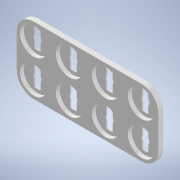
# Autodesk Inventor part: Деталь4
Saved by Autodesk Inventor 2020 (Build 240168000, 168)
## iProperties
Created: 2023-05-30
Part Number: Деталь4
Material: Типовые
Document SubType Name: Modeling
Designer: Qwellert
Density: 1 g/cm^3
Appearance: По умолчанию
Author: Qwellert
Autodesk Inventor part; units mm, degrees
ref_plane "YZ Plane" through (0, 0, 0) normal (1, 0, 0) x (0, 1, 0)
ref_plane "XZ Plane" through (0, 0, 0) normal (0, 1, 0) x (-1, 0, 0)
ref_plane "XY Plane" through (0, 0, 0) normal (0, 0, 1) x (1, 0, 0)
sketch "Эскиз1" plane through (0, 0, 0) normal (0, 0, 1) x (1, 0, 0)
  circle A0 centre (0, 0) radius 13.8038 projected
  arc A1 (3.05, 9.7271) -> (-3.05, 9.7271) centre (0, 0) ccw projected
  line L0 (3.05, 9.7271) -> (3.05, 2.51) projected
  arc A2 (3.05, -2.51) -> (3.05, 2.51) centre (0, 0) ccw projected
  line L1 (3.05, -2.51) -> (3.05, -9.7271) projected
  arc A3 (-3.05, -9.7271) -> (3.05, -9.7271) centre (0, 0) ccw projected
  line L2 (-3.05, -9.7271) -> (-3.05, -2.51) projected
  arc A4 (-3.05, 2.51) -> (-3.05, -2.51) centre (0, 0) ccw projected
  line L3 (-3.05, 2.51) -> (-3.05, 9.7271) projected
  arc A5 (-3.05, 2.51) -> (-3.05, -2.51) centre (0, 0) ccw
  line L4 (-3.05, -2.51) -> (-3.05, -9.7271)
  arc A6 (-3.05, -9.7271) -> (3.05, -9.7271) centre (0, 0) ccw
  line L5 (3.05, -9.7271) -> (3.05, -2.51)
  arc A7 (3.05, -2.51) -> (3.05, 2.51) centre (0, 0) ccw
  line L6 (3.05, 2.51) -> (3.05, 9.7271)
  arc A8 (3.05, 9.7271) -> (-3.05, 9.7271) centre (0, 0) ccw
  line L7 (-3.05, 9.7271) -> (-3.05, 2.51)
  circle A9 centre (0, 0) radius 13.8038
  arc A10 (-3.05, -31.3679) -> (-3.05, -36.3879) centre (0, -33.8779) ccw
  line L8 (-3.05, -36.3879) -> (-3.05, -43.605)
  arc A11 (-3.05, -43.605) -> (3.05, -43.605) centre (0, -33.8779) ccw
  line L9 (3.05, -43.605) -> (3.05, -36.3879)
  arc A12 (3.05, -36.3879) -> (3.05, -31.3679) centre (0, -33.8779) ccw
  line L10 (3.05, -31.3679) -> (3.05, -24.1507)
  arc A13 (3.05, -24.1507) -> (-3.05, -24.1507) centre (0, -33.8779) ccw
  line L11 (-3.05, -24.1507) -> (-3.05, -31.3679)
  circle A14 centre (0, -33.8779) radius 13.8038
  arc A15 (-39.3128, 2.51) -> (-39.3128, -2.51) centre (-36.2628, 0) ccw
  line L12 (-39.3128, -2.51) -> (-39.3128, -9.7271)
  arc A16 (-39.3128, -9.7271) -> (-33.2128, -9.7271) centre (-36.2628, 0) ccw
  line L13 (-33.2128, -9.7271) -> (-33.2128, -2.51)
  arc A17 (-33.2128, -2.51) -> (-33.2128, 2.51) centre (-36.2628, 0) ccw
  line L14 (-33.2128, 2.51) -> (-33.2128, 9.7271)
  arc A18 (-33.2128, 9.7271) -> (-39.3128, 9.7271) centre (-36.2628, 0) ccw
  line L15 (-39.3128, 9.7271) -> (-39.3128, 2.51)
  circle A19 centre (-36.2628, 0) radius 13.8038
  circle A20 centre (-36.2628, -33.8779) radius 13.8038
  line L16 (-33.2128, -43.605) -> (-33.2128, -36.3879)
  arc A21 (-39.3128, -43.605) -> (-33.2128, -43.605) centre (-36.2628, -33.8779) ccw
  line L17 (-39.3128, -36.3879) -> (-39.3128, -43.605)
  arc A22 (-39.3128, -31.3679) -> (-39.3128, -36.3879) centre (-36.2628, -33.8779) ccw
  arc A23 (-33.2128, -36.3879) -> (-33.2128, -31.3679) centre (-36.2628, -33.8779) ccw
  line L18 (-33.2128, -31.3679) -> (-33.2128, -24.1507)
  arc A24 (-33.2128, -24.1507) -> (-39.3128, -24.1507) centre (-36.2628, -33.8779) ccw
  line L19 (-39.3128, -24.1507) -> (-39.3128, -31.3679)
  arc A25 (-75.5758, 2.51) -> (-75.5758, -2.51) centre (-72.5258, 0) ccw
  line L20 (-75.5758, -2.51) -> (-75.5758, -9.7271)
  arc A26 (-75.5758, -9.7271) -> (-69.4758, -9.7271) centre (-72.5258, 0) ccw
  line L21 (-69.4758, -9.7271) -> (-69.4758, -2.51)
  arc A27 (-69.4758, -2.51) -> (-69.4758, 2.51) centre (-72.5258, 0) ccw
  line L22 (-69.4758, 2.51) -> (-69.4758, 9.7271)
  arc A28 (-69.4758, 9.7271) -> (-75.5758, 9.7271) centre (-72.5258, 0) ccw
  line L23 (-75.5758, 9.7271) -> (-75.5758, 2.51)
  circle A29 centre (-72.5258, 0) radius 13.8038
  circle A30 centre (-72.5258, -33.8779) radius 13.8038
  line L24 (-69.4758, -43.605) -> (-69.4758, -36.3879)
  arc A31 (-75.5758, -43.605) -> (-69.4758, -43.605) centre (-72.5258, -33.8779) ccw
  line L25 (-75.5758, -36.3879) -> (-75.5758, -43.605)
  arc A32 (-75.5758, -31.3679) -> (-75.5758, -36.3879) centre (-72.5258, -33.8779) ccw
  arc A33 (-69.4758, -36.3879) -> (-69.4758, -31.3679) centre (-72.5258, -33.8779) ccw
  line L26 (-69.4758, -31.3679) -> (-69.4758, -24.1507)
  arc A34 (-69.4758, -24.1507) -> (-75.5758, -24.1507) centre (-72.5258, -33.8779) ccw
  line L27 (-75.5758, -24.1507) -> (-75.5758, -31.3679)
  circle A35 centre (-108.7886, 0) radius 13.8038
  line L28 (-105.7386, -9.7271) -> (-105.7386, -2.51)
  arc A36 (-111.8386, -9.7271) -> (-105.7386, -9.7271) centre (-108.7886, 0) ccw
  line L29 (-111.8386, -2.51) -> (-111.8386, -9.7271)
  arc A37 (-111.8386, 2.51) -> (-111.8386, -2.51) centre (-108.7886, 0) ccw
  arc A38 (-105.7386, -2.51) -> (-105.7386, 2.51) centre (-108.7886, 0) ccw
  line L30 (-105.7386, 2.51) -> (-105.7386, 9.7271)
  arc A39 (-105.7386, 9.7271) -> (-111.8386, 9.7271) centre (-108.7886, 0) ccw
  line L31 (-111.8386, 9.7271) -> (-111.8386, 2.51)
  circle A40 centre (-108.7886, -33.8779) radius 13.8038
  line L32 (-105.7386, -31.3679) -> (-105.7386, -24.1507)
  arc A41 (-105.7386, -36.3879) -> (-105.7386, -31.3679) centre (-108.7886, -33.8779) ccw
  line L33 (-105.7386, -43.605) -> (-105.7386, -36.3879)
  arc A42 (-111.8386, -43.605) -> (-105.7386, -43.605) centre (-108.7886, -33.8779) ccw
  line L34 (-111.8386, -36.3879) -> (-111.8386, -43.605)
  line L35 (-111.8386, -24.1507) -> (-111.8386, -31.3679)
  arc A43 (-105.7386, -24.1507) -> (-111.8386, -24.1507) centre (-108.7886, -33.8779) ccw
  arc A44 (-111.8386, -31.3679) -> (-111.8386, -36.3879) centre (-108.7886, -33.8779) ccw
  constraints: 64 end point, 64 point on circle, 40 centre point, 32 vertical, 80 other
extrude "Выдавливание1" add sketch "Эскиз1" along normal blind 1
sketch "Эскиз2" plane through (0, -33.8779, 0) normal (0, 0, -1) x (-1, 0, 0)
  arc A0 (-3.05, 36.3879) -> (-3.05, 31.3679) centre (0, 33.8779) ccw projected
  circle A1 centre (0, 33.8779) radius 16.8507
  circle A2 centre (0, 0) radius 13.8038 projected
  arc A3 (33.2128, -9.7271) -> (39.3128, -9.7271) centre (36.2628, 0) ccw projected
  line L0 (39.3128, -9.7271) -> (39.3128, -2.51) projected
  arc A4 (39.3128, -2.51) -> (39.3128, 2.51) centre (36.2628, 0) ccw projected
  line L1 (39.3128, 2.51) -> (39.3128, 9.7271) projected
  arc A5 (39.3128, 9.7271) -> (33.2128, 9.7271) centre (36.2628, 0) ccw projected
  line L2 (33.2128, 9.7271) -> (33.2128, 2.51) projected
  arc A6 (33.2128, 2.51) -> (33.2128, -2.51) centre (36.2628, 0) ccw projected
  line L3 (33.2128, -2.51) -> (33.2128, -9.7271) projected
  circle A7 centre (36.2628, 0) radius 13.8038 projected
  line L4 (111.8386, 2.51) -> (111.8386, 9.7271) projected
  arc A8 (111.8386, 9.7271) -> (105.7386, 9.7271) centre (108.7886, 0) ccw projected
  line L5 (105.7386, 9.7271) -> (105.7386, 2.51) projected
  arc A9 (105.7386, 2.51) -> (105.7386, -2.51) centre (108.7886, 0) ccw projected
  line L6 (105.7386, -2.51) -> (105.7386, -9.7271) projected
  arc A10 (105.7386, -9.7271) -> (111.8386, -9.7271) centre (108.7886, 0) ccw projected
  line L7 (111.8386, -9.7271) -> (111.8386, -2.51) projected
  arc A11 (111.8386, -2.51) -> (111.8386, 2.51) centre (108.7886, 0) ccw projected
  circle A12 centre (108.7886, 0) radius 13.8038 projected
  line L8 (69.4758, 31.3679) -> (69.4758, 24.1507) projected
  arc A13 (69.4758, 24.1507) -> (75.5758, 24.1507) centre (72.5258, 33.8779) ccw projected
  line L9 (75.5758, 24.1507) -> (75.5758, 31.3679) projected
  arc A14 (75.5758, 31.3679) -> (75.5758, 36.3879) centre (72.5258, 33.8779) ccw projected
  line L10 (75.5758, 36.3879) -> (75.5758, 43.605) projected
  arc A15 (75.5758, 43.605) -> (69.4758, 43.605) centre (72.5258, 33.8779) ccw projected
  line L11 (69.4758, 43.605) -> (69.4758, 36.3879) projected
  arc A16 (69.4758, 36.3879) -> (69.4758, 31.3679) centre (72.5258, 33.8779) ccw projected
  circle A17 centre (72.5258, 33.8779) radius 13.8038 projected
  arc A18 (-3.05, 2.51) -> (-3.05, -2.51) centre (0, 0) ccw projected
  line L12 (-3.05, -2.51) -> (-3.05, -9.7271) projected
  arc A19 (-3.05, -9.7271) -> (3.05, -9.7271) centre (0, 0) ccw projected
  line L13 (3.05, -9.7271) -> (3.05, -2.51) projected
  arc A20 (3.05, -2.51) -> (3.05, 2.51) centre (0, 0) ccw projected
  line L14 (3.05, 2.51) -> (3.05, 9.7271) projected
  arc A21 (3.05, 9.7271) -> (-3.05, 9.7271) centre (0, 0) ccw projected
  line L15 (-3.05, 9.7271) -> (-3.05, 2.51) projected
  circle A22 centre (0, 0) radius 13.8038 projected
  arc A23 (33.2128, 24.1507) -> (39.3128, 24.1507) centre (36.2628, 33.8779) ccw projected
  line L16 (39.3128, 24.1507) -> (39.3128, 31.3679) projected
  arc A24 (39.3128, 31.3679) -> (39.3128, 36.3879) centre (36.2628, 33.8779) ccw projected
  line L17 (39.3128, 36.3879) -> (39.3128, 43.605) projected
  arc A25 (39.3128, 43.605) -> (33.2128, 43.605) centre (36.2628, 33.8779) ccw projected
  line L18 (33.2128, 43.605) -> (33.2128, 36.3879) projected
  arc A26 (33.2128, 36.3879) -> (33.2128, 31.3679) centre (36.2628, 33.8779) ccw projected
  line L19 (33.2128, 31.3679) -> (33.2128, 24.1507) projected
  circle A27 centre (36.2628, 33.8779) radius 13.8038 projected
  line L20 (105.7386, 31.3679) -> (105.7386, 24.1507) projected
  arc A28 (105.7386, 24.1507) -> (111.8386, 24.1507) centre (108.7886, 33.8779) ccw projected
  line L21 (111.8386, 24.1507) -> (111.8386, 31.3679) projected
  arc A29 (111.8386, 31.3679) -> (111.8386, 36.3879) centre (108.7886, 33.8779) ccw projected
  line L22 (111.8386, 36.3879) -> (111.8386, 43.605) projected
  arc A30 (111.8386, 43.605) -> (105.7386, 43.605) centre (108.7886, 33.8779) ccw projected
  line L23 (105.7386, 43.605) -> (105.7386, 36.3879) projected
  arc A31 (105.7386, 36.3879) -> (105.7386, 31.3679) centre (108.7886, 33.8779) ccw projected
  circle A32 centre (108.7886, 33.8779) radius 13.8038 projected
  arc A33 (75.5758, -2.51) -> (75.5758, 2.51) centre (72.5258, 0) ccw projected
  line L24 (75.5758, 2.51) -> (75.5758, 9.7271) projected
  arc A34 (75.5758, 9.7271) -> (69.4758, 9.7271) centre (72.5258, 0) ccw projected
  line L25 (69.4758, 9.7271) -> (69.4758, 2.51) projected
  arc A35 (69.4758, 2.51) -> (69.4758, -2.51) centre (72.5258, 0) ccw projected
  line L26 (69.4758, -2.51) -> (69.4758, -9.7271) projected
  arc A36 (69.4758, -9.7271) -> (75.5758, -9.7271) centre (72.5258, 0) ccw projected
  line L27 (75.5758, -9.7271) -> (75.5758, -2.51) projected
  circle A37 centre (72.5258, 0) radius 13.8038 projected
  line L28 (3.05, 24.1507) -> (3.05, 31.3679) projected
  arc A38 (3.05, 31.3679) -> (3.05, 36.3879) centre (0, 33.8779) ccw projected
  line L29 (3.05, 36.3879) -> (3.05, 43.605) projected
  arc A39 (3.05, 43.605) -> (-3.05, 43.605) centre (0, 33.8779) ccw projected
  line L30 (-3.05, 43.605) -> (-3.05, 36.3879) projected
  arc A40 (-3.05, 36.3879) -> (-3.05, 31.3679) centre (0, 33.8779) ccw projected
  line L31 (-3.05, 31.3679) -> (-3.05, 24.1507) projected
  arc A41 (-3.05, 24.1507) -> (3.05, 24.1507) centre (0, 33.8779) ccw projected
  circle A42 centre (0, 33.8779) radius 13.8038 projected
  circle A43 centre (0, 0) radius 16.8507
  circle A44 centre (36.2628, 0) radius 16.8507
  circle A45 centre (36.2628, 33.8779) radius 16.8507
  circle A46 centre (72.5258, 33.8779) radius 16.8507
  circle A47 centre (72.5258, 0) radius 16.8507
  circle A48 centre (108.7886, 0) radius 16.8507
  circle A49 centre (108.7886, 33.8779) radius 16.8507
  arc A50 (3.05, 31.3679) -> (3.05, 36.3879) centre (0, 33.8779) ccw
  line L32 (3.05, 36.3879) -> (3.05, 43.605)
  arc A51 (3.05, 43.605) -> (-3.05, 43.605) centre (0, 33.8779) ccw
  line L33 (-3.05, 43.605) -> (-3.05, 36.3879)
  arc A52 (-3.05, 36.3879) -> (-3.05, 31.3679) centre (0, 33.8779) ccw
  line L34 (-3.05, 31.3679) -> (-3.05, 24.1507)
  arc A53 (-3.05, 24.1507) -> (3.05, 24.1507) centre (0, 33.8779) ccw
  line L35 (3.05, 24.1507) -> (3.05, 31.3679)
  circle A54 centre (0, 33.8779) radius 13.8038
  arc A55 (33.2128, -9.7271) -> (39.3128, -9.7271) centre (36.2628, 0) ccw projected
  line L36 (39.3128, -9.7271) -> (39.3128, -2.51) projected
  arc A56 (39.3128, -2.51) -> (39.3128, 2.51) centre (36.2628, 0) ccw projected
  line L37 (39.3128, 2.51) -> (39.3128, 9.7271) projected
  arc A57 (39.3128, 9.7271) -> (33.2128, 9.7271) centre (36.2628, 0) ccw projected
  line L38 (33.2128, 9.7271) -> (33.2128, 2.51) projected
  arc A58 (33.2128, 2.51) -> (33.2128, -2.51) centre (36.2628, 0) ccw projected
  line L39 (33.2128, -2.51) -> (33.2128, -9.7271) projected
  circle A59 centre (36.2628, 0) radius 13.8038 projected
  line L40 (111.8386, 2.51) -> (111.8386, 9.7271) projected
  arc A60 (111.8386, 9.7271) -> (105.7386, 9.7271) centre (108.7886, 0) ccw projected
  line L41 (105.7386, 9.7271) -> (105.7386, 2.51) projected
  arc A61 (105.7386, 2.51) -> (105.7386, -2.51) centre (108.7886, 0) ccw projected
  line L42 (105.7386, -2.51) -> (105.7386, -9.7271) projected
  arc A62 (105.7386, -9.7271) -> (111.8386, -9.7271) centre (108.7886, 0) ccw projected
  line L43 (111.8386, -9.7271) -> (111.8386, -2.51) projected
  arc A63 (111.8386, -2.51) -> (111.8386, 2.51) centre (108.7886, 0) ccw projected
  circle A64 centre (108.7886, 0) radius 13.8038 projected
  line L44 (69.4758, 31.3679) -> (69.4758, 24.1507) projected
  arc A65 (69.4758, 24.1507) -> (75.5758, 24.1507) centre (72.5258, 33.8779) ccw projected
  line L45 (75.5758, 24.1507) -> (75.5758, 31.3679) projected
  arc A66 (75.5758, 31.3679) -> (75.5758, 36.3879) centre (72.5258, 33.8779) ccw projected
  line L46 (75.5758, 36.3879) -> (75.5758, 43.605) projected
  arc A67 (75.5758, 43.605) -> (69.4758, 43.605) centre (72.5258, 33.8779) ccw projected
  line L47 (69.4758, 43.605) -> (69.4758, 36.3879) projected
  arc A68 (69.4758, 36.3879) -> (69.4758, 31.3679) centre (72.5258, 33.8779) ccw projected
  circle A69 centre (72.5258, 33.8779) radius 13.8038 projected
  arc A70 (-3.05, 2.51) -> (-3.05, -2.51) centre (0, 0) ccw projected
  line L48 (-3.05, -2.51) -> (-3.05, -9.7271) projected
  arc A71 (-3.05, -9.7271) -> (3.05, -9.7271) centre (0, 0) ccw projected
  line L49 (3.05, -9.7271) -> (3.05, -2.51) projected
  arc A72 (3.05, -2.51) -> (3.05, 2.51) centre (0, 0) ccw projected
  line L50 (3.05, 2.51) -> (3.05, 9.7271) projected
  arc A73 (3.05, 9.7271) -> (-3.05, 9.7271) centre (0, 0) ccw projected
  line L51 (-3.05, 9.7271) -> (-3.05, 2.51) projected
  circle A74 centre (0, 0) radius 13.8038 projected
  arc A75 (33.2128, 24.1507) -> (39.3128, 24.1507) centre (36.2628, 33.8779) ccw projected
  line L52 (39.3128, 24.1507) -> (39.3128, 31.3679) projected
  arc A76 (39.3128, 31.3679) -> (39.3128, 36.3879) centre (36.2628, 33.8779) ccw projected
  line L53 (39.3128, 36.3879) -> (39.3128, 43.605) projected
  arc A77 (39.3128, 43.605) -> (33.2128, 43.605) centre (36.2628, 33.8779) ccw projected
  line L54 (33.2128, 43.605) -> (33.2128, 36.3879) projected
  arc A78 (33.2128, 36.3879) -> (33.2128, 31.3679) centre (36.2628, 33.8779) ccw projected
  line L55 (33.2128, 31.3679) -> (33.2128, 24.1507) projected
  circle A79 centre (36.2628, 33.8779) radius 13.8038 projected
  line L56 (105.7386, 31.3679) -> (105.7386, 24.1507) projected
  arc A80 (105.7386, 24.1507) -> (111.8386, 24.1507) centre (108.7886, 33.8779) ccw projected
  line L57 (111.8386, 24.1507) -> (111.8386, 31.3679) projected
  arc A81 (111.8386, 31.3679) -> (111.8386, 36.3879) centre (108.7886, 33.8779) ccw projected
  line L58 (111.8386, 36.3879) -> (111.8386, 43.605) projected
  arc A82 (111.8386, 43.605) -> (105.7386, 43.605) centre (108.7886, 33.8779) ccw projected
  line L59 (105.7386, 43.605) -> (105.7386, 36.3879) projected
  arc A83 (105.7386, 36.3879) -> (105.7386, 31.3679) centre (108.7886, 33.8779) ccw projected
  circle A84 centre (108.7886, 33.8779) radius 13.8038 projected
  arc A85 (75.5758, -2.51) -> (75.5758, 2.51) centre (72.5258, 0) ccw projected
  line L60 (75.5758, 2.51) -> (75.5758, 9.7271) projected
  arc A86 (75.5758, 9.7271) -> (69.4758, 9.7271) centre (72.5258, 0) ccw projected
  line L61 (69.4758, 9.7271) -> (69.4758, 2.51) projected
  arc A87 (69.4758, 2.51) -> (69.4758, -2.51) centre (72.5258, 0) ccw projected
  line L62 (69.4758, -2.51) -> (69.4758, -9.7271) projected
  arc A88 (69.4758, -9.7271) -> (75.5758, -9.7271) centre (72.5258, 0) ccw projected
  line L63 (75.5758, -9.7271) -> (75.5758, -2.51) projected
  circle A89 centre (72.5258, 0) radius 13.8038 projected
  line L64 (3.05, 24.1507) -> (3.05, 31.3679) projected
  arc A90 (3.05, 31.3679) -> (3.05, 36.3879) centre (0, 33.8779) ccw projected
  line L65 (3.05, 36.3879) -> (3.05, 43.605) projected
  arc A91 (3.05, 43.605) -> (-3.05, 43.605) centre (0, 33.8779) ccw projected
  line L66 (-3.05, 43.605) -> (-3.05, 36.3879) projected
  arc A92 (-3.05, 36.3879) -> (-3.05, 31.3679) centre (0, 33.8779) ccw projected
  line L67 (-3.05, 31.3679) -> (-3.05, 24.1507) projected
  arc A93 (-3.05, 24.1507) -> (3.05, 24.1507) centre (0, 33.8779) ccw projected
  circle A94 centre (0, 33.8779) radius 13.8038 projected
  arc A95 (33.2128, -9.7271) -> (39.3128, -9.7271) centre (36.2628, 0) ccw projected
  line L68 (39.3128, -9.7271) -> (39.3128, -2.51) projected
  arc A96 (39.3128, -2.51) -> (39.3128, 2.51) centre (36.2628, 0) ccw projected
  line L69 (39.3128, 2.51) -> (39.3128, 9.7271) projected
  arc A97 (39.3128, 9.7271) -> (33.2128, 9.7271) centre (36.2628, 0) ccw projected
  line L70 (33.2128, 9.7271) -> (33.2128, 2.51) projected
  arc A98 (33.2128, 2.51) -> (33.2128, -2.51) centre (36.2628, 0) ccw projected
  line L71 (33.2128, -2.51) -> (33.2128, -9.7271) projected
  circle A99 centre (36.2628, 0) radius 13.8038 projected
  line L72 (111.8386, 2.51) -> (111.8386, 9.7271) projected
  arc A100 (111.8386, 9.7271) -> (105.7386, 9.7271) centre (108.7886, 0) ccw projected
  line L73 (105.7386, 9.7271) -> (105.7386, 2.51) projected
  arc A101 (105.7386, 2.51) -> (105.7386, -2.51) centre (108.7886, 0) ccw projected
  line L74 (105.7386, -2.51) -> (105.7386, -9.7271) projected
  arc A102 (105.7386, -9.7271) -> (111.8386, -9.7271) centre (108.7886, 0) ccw projected
  line L75 (111.8386, -9.7271) -> (111.8386, -2.51) projected
  arc A103 (111.8386, -2.51) -> (111.8386, 2.51) centre (108.7886, 0) ccw projected
  circle A104 centre (108.7886, 0) radius 13.8038 projected
  line L76 (69.4758, 31.3679) -> (69.4758, 24.1507) projected
  arc A105 (69.4758, 24.1507) -> (75.5758, 24.1507) centre (72.5258, 33.8779) ccw projected
  line L77 (75.5758, 24.1507) -> (75.5758, 31.3679) projected
  arc A106 (75.5758, 31.3679) -> (75.5758, 36.3879) centre (72.5258, 33.8779) ccw projected
  line L78 (75.5758, 36.3879) -> (75.5758, 43.605) projected
  arc A107 (75.5758, 43.605) -> (69.4758, 43.605) centre (72.5258, 33.8779) ccw projected
  line L79 (69.4758, 43.605) -> (69.4758, 36.3879) projected
  arc A108 (69.4758, 36.3879) -> (69.4758, 31.3679) centre (72.5258, 33.8779) ccw projected
  circle A109 centre (72.5258, 33.8779) radius 13.8038 projected
  arc A110 (-3.05, 2.51) -> (-3.05, -2.51) centre (0, 0) ccw projected
  line L80 (-3.05, -2.51) -> (-3.05, -9.7271) projected
  arc A111 (-3.05, -9.7271) -> (3.05, -9.7271) centre (0, 0) ccw projected
  line L81 (3.05, -9.7271) -> (3.05, -2.51) projected
  arc A112 (3.05, -2.51) -> (3.05, 2.51) centre (0, 0) ccw projected
  line L82 (3.05, 2.51) -> (3.05, 9.7271) projected
  arc A113 (3.05, 9.7271) -> (-3.05, 9.7271) centre (0, 0) ccw projected
  line L83 (-3.05, 9.7271) -> (-3.05, 2.51) projected
  circle A114 centre (0, 0) radius 13.8038 projected
  arc A115 (33.2128, 24.1507) -> (39.3128, 24.1507) centre (36.2628, 33.8779) ccw projected
  line L84 (39.3128, 24.1507) -> (39.3128, 31.3679) projected
  arc A116 (39.3128, 31.3679) -> (39.3128, 36.3879) centre (36.2628, 33.8779) ccw projected
  line L85 (39.3128, 36.3879) -> (39.3128, 43.605) projected
  arc A117 (39.3128, 43.605) -> (33.2128, 43.605) centre (36.2628, 33.8779) ccw projected
  line L86 (33.2128, 43.605) -> (33.2128, 36.3879) projected
  arc A118 (33.2128, 36.3879) -> (33.2128, 31.3679) centre (36.2628, 33.8779) ccw projected
  line L87 (33.2128, 31.3679) -> (33.2128, 24.1507) projected
  circle A119 centre (36.2628, 33.8779) radius 13.8038 projected
  line L88 (105.7386, 31.3679) -> (105.7386, 24.1507) projected
  arc A120 (105.7386, 24.1507) -> (111.8386, 24.1507) centre (108.7886, 33.8779) ccw projected
  line L89 (111.8386, 24.1507) -> (111.8386, 31.3679) projected
  arc A121 (111.8386, 31.3679) -> (111.8386, 36.3879) centre (108.7886, 33.8779) ccw projected
  line L90 (111.8386, 36.3879) -> (111.8386, 43.605) projected
  arc A122 (111.8386, 43.605) -> (105.7386, 43.605) centre (108.7886, 33.8779) ccw projected
  line L91 (105.7386, 43.605) -> (105.7386, 36.3879) projected
  arc A123 (105.7386, 36.3879) -> (105.7386, 31.3679) centre (108.7886, 33.8779) ccw projected
  circle A124 centre (108.7886, 33.8779) radius 13.8038 projected
  arc A125 (75.5758, -2.51) -> (75.5758, 2.51) centre (72.5258, 0) ccw projected
  line L92 (75.5758, 2.51) -> (75.5758, 9.7271) projected
  arc A126 (75.5758, 9.7271) -> (69.4758, 9.7271) centre (72.5258, 0) ccw projected
  line L93 (69.4758, 9.7271) -> (69.4758, 2.51) projected
  arc A127 (69.4758, 2.51) -> (69.4758, -2.51) centre (72.5258, 0) ccw projected
  line L94 (69.4758, -2.51) -> (69.4758, -9.7271) projected
  arc A128 (69.4758, -9.7271) -> (75.5758, -9.7271) centre (72.5258, 0) ccw projected
  line L95 (75.5758, -9.7271) -> (75.5758, -2.51) projected
  circle A129 centre (72.5258, 0) radius 13.8038 projected
  line L96 (3.05, 24.1507) -> (3.05, 31.3679) projected
  arc A130 (3.05, 31.3679) -> (3.05, 36.3879) centre (0, 33.8779) ccw projected
  line L97 (3.05, 36.3879) -> (3.05, 43.605) projected
  arc A131 (3.05, 43.605) -> (-3.05, 43.605) centre (0, 33.8779) ccw projected
  line L98 (-3.05, 43.605) -> (-3.05, 36.3879) projected
  arc A132 (-3.05, 36.3879) -> (-3.05, 31.3679) centre (0, 33.8779) ccw projected
  line L99 (-3.05, 31.3679) -> (-3.05, 24.1507) projected
  arc A133 (-3.05, 24.1507) -> (3.05, 24.1507) centre (0, 33.8779) ccw projected
  circle A134 centre (0, 33.8779) radius 13.8038 projected
  arc A135 (33.2128, -9.7271) -> (39.3128, -9.7271) centre (36.2628, 0) ccw projected
  line L100 (39.3128, -9.7271) -> (39.3128, -2.51) projected
  arc A136 (39.3128, -2.51) -> (39.3128, 2.51) centre (36.2628, 0) ccw projected
  line L101 (39.3128, 2.51) -> (39.3128, 9.7271) projected
  arc A137 (39.3128, 9.7271) -> (33.2128, 9.7271) centre (36.2628, 0) ccw projected
  line L102 (33.2128, 9.7271) -> (33.2128, 2.51) projected
  arc A138 (33.2128, 2.51) -> (33.2128, -2.51) centre (36.2628, 0) ccw projected
  line L103 (33.2128, -2.51) -> (33.2128, -9.7271) projected
  circle A139 centre (36.2628, 0) radius 13.8038 projected
  line L104 (111.8386, 2.51) -> (111.8386, 9.7271) projected
  arc A140 (111.8386, 9.7271) -> (105.7386, 9.7271) centre (108.7886, 0) ccw projected
  line L105 (105.7386, 9.7271) -> (105.7386, 2.51) projected
  arc A141 (105.7386, 2.51) -> (105.7386, -2.51) centre (108.7886, 0) ccw projected
  line L106 (105.7386, -2.51) -> (105.7386, -9.7271) projected
  arc A142 (105.7386, -9.7271) -> (111.8386, -9.7271) centre (108.7886, 0) ccw projected
  line L107 (111.8386, -9.7271) -> (111.8386, -2.51) projected
  arc A143 (111.8386, -2.51) -> (111.8386, 2.51) centre (108.7886, 0) ccw projected
  circle A144 centre (108.7886, 0) radius 13.8038 projected
  line L108 (69.4758, 31.3679) -> (69.4758, 24.1507) projected
  arc A145 (69.4758, 24.1507) -> (75.5758, 24.1507) centre (72.5258, 33.8779) ccw projected
  line L109 (75.5758, 24.1507) -> (75.5758, 31.3679) projected
  arc A146 (75.5758, 31.3679) -> (75.5758, 36.3879) centre (72.5258, 33.8779) ccw projected
  line L110 (75.5758, 36.3879) -> (75.5758, 43.605) projected
  arc A147 (75.5758, 43.605) -> (69.4758, 43.605) centre (72.5258, 33.8779) ccw projected
  line L111 (69.4758, 43.605) -> (69.4758, 36.3879) projected
  arc A148 (69.4758, 36.3879) -> (69.4758, 31.3679) centre (72.5258, 33.8779) ccw projected
  circle A149 centre (72.5258, 33.8779) radius 13.8038 projected
  arc A150 (-3.05, 2.51) -> (-3.05, -2.51) centre (0, 0) ccw projected
  line L112 (-3.05, -2.51) -> (-3.05, -9.7271) projected
  arc A151 (-3.05, -9.7271) -> (3.05, -9.7271) centre (0, 0) ccw projected
  line L113 (3.05, -9.7271) -> (3.05, -2.51) projected
  arc A152 (3.05, -2.51) -> (3.05, 2.51) centre (0, 0) ccw projected
  line L114 (3.05, 2.51) -> (3.05, 9.7271) projected
  arc A153 (3.05, 9.7271) -> (-3.05, 9.7271) centre (0, 0) ccw projected
  line L115 (-3.05, 9.7271) -> (-3.05, 2.51) projected
  circle A154 centre (0, 0) radius 13.8038 projected
  arc A155 (33.2128, 24.1507) -> (39.3128, 24.1507) centre (36.2628, 33.8779) ccw projected
  line L116 (39.3128, 24.1507) -> (39.3128, 31.3679) projected
  arc A156 (39.3128, 31.3679) -> (39.3128, 36.3879) centre (36.2628, 33.8779) ccw projected
  line L117 (39.3128, 36.3879) -> (39.3128, 43.605) projected
  arc A157 (39.3128, 43.605) -> (33.2128, 43.605) centre (36.2628, 33.8779) ccw projected
  line L118 (33.2128, 43.605) -> (33.2128, 36.3879) projected
  arc A158 (33.2128, 36.3879) -> (33.2128, 31.3679) centre (36.2628, 33.8779) ccw projected
  line L119 (33.2128, 31.3679) -> (33.2128, 24.1507) projected
  circle A159 centre (36.2628, 33.8779) radius 13.8038 projected
  line L120 (105.7386, 31.3679) -> (105.7386, 24.1507) projected
  arc A160 (105.7386, 24.1507) -> (111.8386, 24.1507) centre (108.7886, 33.8779) ccw projected
  line L121 (111.8386, 24.1507) -> (111.8386, 31.3679) projected
  arc A161 (111.8386, 31.3679) -> (111.8386, 36.3879) centre (108.7886, 33.8779) ccw projected
  line L122 (111.8386, 36.3879) -> (111.8386, 43.605) projected
  arc A162 (111.8386, 43.605) -> (105.7386, 43.605) centre (108.7886, 33.8779) ccw projected
  line L123 (105.7386, 43.605) -> (105.7386, 36.3879) projected
  arc A163 (105.7386, 36.3879) -> (105.7386, 31.3679) centre (108.7886, 33.8779) ccw projected
  circle A164 centre (108.7886, 33.8779) radius 13.8038 projected
  arc A165 (75.5758, -2.51) -> (75.5758, 2.51) centre (72.5258, 0) ccw projected
  line L124 (75.5758, 2.51) -> (75.5758, 9.7271) projected
  arc A166 (75.5758, 9.7271) -> (69.4758, 9.7271) centre (72.5258, 0) ccw projected
  line L125 (69.4758, 9.7271) -> (69.4758, 2.51) projected
  arc A167 (69.4758, 2.51) -> (69.4758, -2.51) centre (72.5258, 0) ccw projected
  line L126 (69.4758, -2.51) -> (69.4758, -9.7271) projected
  arc A168 (69.4758, -9.7271) -> (75.5758, -9.7271) centre (72.5258, 0) ccw projected
  line L127 (75.5758, -9.7271) -> (75.5758, -2.51) projected
  circle A169 centre (72.5258, 0) radius 13.8038 projected
  line L128 (3.05, 24.1507) -> (3.05, 31.3679) projected
  arc A170 (3.05, 31.3679) -> (3.05, 36.3879) centre (0, 33.8779) ccw projected
  line L129 (3.05, 36.3879) -> (3.05, 43.605) projected
  arc A171 (3.05, 43.605) -> (-3.05, 43.605) centre (0, 33.8779) ccw projected
  line L130 (-3.05, 43.605) -> (-3.05, 36.3879) projected
  arc A172 (-3.05, 36.3879) -> (-3.05, 31.3679) centre (0, 33.8779) ccw projected
  line L131 (-3.05, 31.3679) -> (-3.05, 24.1507) projected
  arc A173 (-3.05, 24.1507) -> (3.05, 24.1507) centre (0, 33.8779) ccw projected
  circle A174 centre (0, 33.8779) radius 13.8038 projected
  arc A175 (33.2128, -9.7271) -> (39.3128, -9.7271) centre (36.2628, 0) ccw projected
  line L132 (39.3128, -9.7271) -> (39.3128, -2.51) projected
  arc A176 (39.3128, -2.51) -> (39.3128, 2.51) centre (36.2628, 0) ccw projected
  line L133 (39.3128, 2.51) -> (39.3128, 9.7271) projected
  arc A177 (39.3128, 9.7271) -> (33.2128, 9.7271) centre (36.2628, 0) ccw projected
  line L134 (33.2128, 9.7271) -> (33.2128, 2.51) projected
  arc A178 (33.2128, 2.51) -> (33.2128, -2.51) centre (36.2628, 0) ccw projected
  line L135 (33.2128, -2.51) -> (33.2128, -9.7271) projected
  circle A179 centre (36.2628, 0) radius 13.8038 projected
  line L136 (111.8386, 2.51) -> (111.8386, 9.7271) projected
  arc A180 (111.8386, 9.7271) -> (105.7386, 9.7271) centre (108.7886, 0) ccw projected
  line L137 (105.7386, 9.7271) -> (105.7386, 2.51) projected
  arc A181 (105.7386, 2.51) -> (105.7386, -2.51) centre (108.7886, 0) ccw projected
  line L138 (105.7386, -2.51) -> (105.7386, -9.7271) projected
  arc A182 (105.7386, -9.7271) -> (111.8386, -9.7271) centre (108.7886, 0) ccw projected
  line L139 (111.8386, -9.7271) -> (111.8386, -2.51) projected
  arc A183 (111.8386, -2.51) -> (111.8386, 2.51) centre (108.7886, 0) ccw projected
  circle A184 centre (108.7886, 0) radius 13.8038 projected
  line L140 (69.4758, 31.3679) -> (69.4758, 24.1507) projected
  arc A185 (69.4758, 24.1507) -> (75.5758, 24.1507) centre (72.5258, 33.8779) ccw projected
  line L141 (75.5758, 24.1507) -> (75.5758, 31.3679) projected
  arc A186 (75.5758, 31.3679) -> (75.5758, 36.3879) centre (72.5258, 33.8779) ccw projected
  line L142 (75.5758, 36.3879) -> (75.5758, 43.605) projected
  arc A187 (75.5758, 43.605) -> (69.4758, 43.605) centre (72.5258, 33.8779) ccw projected
  line L143 (69.4758, 43.605) -> (69.4758, 36.3879) projected
  arc A188 (69.4758, 36.3879) -> (69.4758, 31.3679) centre (72.5258, 33.8779) ccw projected
  circle A189 centre (72.5258, 33.8779) radius 13.8038 projected
  arc A190 (-3.05, 2.51) -> (-3.05, -2.51) centre (0, 0) ccw projected
  line L144 (-3.05, -2.51) -> (-3.05, -9.7271) projected
  arc A191 (-3.05, -9.7271) -> (3.05, -9.7271) centre (0, 0) ccw projected
  line L145 (3.05, -9.7271) -> (3.05, -2.51) projected
  arc A192 (3.05, -2.51) -> (3.05, 2.51) centre (0, 0) ccw projected
  line L146 (3.05, 2.51) -> (3.05, 9.7271) projected
  arc A193 (3.05, 9.7271) -> (-3.05, 9.7271) centre (0, 0) ccw projected
  line L147 (-3.05, 9.7271) -> (-3.05, 2.51) projected
  circle A194 centre (0, 0) radius 13.8038 projected
  arc A195 (33.2128, 24.1507) -> (39.3128, 24.1507) centre (36.2628, 33.8779) ccw projected
  line L148 (39.3128, 24.1507) -> (39.3128, 31.3679) projected
  arc A196 (39.3128, 31.3679) -> (39.3128, 36.3879) centre (36.2628, 33.8779) ccw projected
  line L149 (39.3128, 36.3879) -> (39.3128, 43.605) projected
  arc A197 (39.3128, 43.605) -> (33.2128, 43.605) centre (36.2628, 33.8779) ccw projected
  line L150 (33.2128, 43.605) -> (33.2128, 36.3879) projected
  arc A198 (33.2128, 36.3879) -> (33.2128, 31.3679) centre (36.2628, 33.8779) ccw projected
  line L151 (33.2128, 31.3679) -> (33.2128, 24.1507) projected
  circle A199 centre (36.2628, 33.8779) radius 13.8038 projected
  line L152 (105.7386, 31.3679) -> (105.7386, 24.1507) projected
  arc A200 (105.7386, 24.1507) -> (111.8386, 24.1507) centre (108.7886, 33.8779) ccw projected
  line L153 (111.8386, 24.1507) -> (111.8386, 31.3679) projected
  arc A201 (111.8386, 31.3679) -> (111.8386, 36.3879) centre (108.7886, 33.8779) ccw projected
  line L154 (111.8386, 36.3879) -> (111.8386, 43.605) projected
  arc A202 (111.8386, 43.605) -> (105.7386, 43.605) centre (108.7886, 33.8779) ccw projected
  line L155 (105.7386, 43.605) -> (105.7386, 36.3879) projected
  arc A203 (105.7386, 36.3879) -> (105.7386, 31.3679) centre (108.7886, 33.8779) ccw projected
  circle A204 centre (108.7886, 33.8779) radius 13.8038 projected
  arc A205 (75.5758, -2.51) -> (75.5758, 2.51) centre (72.5258, 0) ccw projected
  line L156 (75.5758, 2.51) -> (75.5758, 9.7271) projected
  arc A206 (75.5758, 9.7271) -> (69.4758, 9.7271) centre (72.5258, 0) ccw projected
  line L157 (69.4758, 9.7271) -> (69.4758, 2.51) projected
  arc A207 (69.4758, 2.51) -> (69.4758, -2.51) centre (72.5258, 0) ccw projected
  line L158 (69.4758, -2.51) -> (69.4758, -9.7271) projected
  arc A208 (69.4758, -9.7271) -> (75.5758, -9.7271) centre (72.5258, 0) ccw projected
  line L159 (75.5758, -9.7271) -> (75.5758, -2.51) projected
  circle A209 centre (72.5258, 0) radius 13.8038 projected
  line L160 (3.05, 24.1507) -> (3.05, 31.3679) projected
  arc A210 (3.05, 31.3679) -> (3.05, 36.3879) centre (0, 33.8779) ccw projected
  line L161 (3.05, 36.3879) -> (3.05, 43.605) projected
  arc A211 (3.05, 43.605) -> (-3.05, 43.605) centre (0, 33.8779) ccw projected
  line L162 (-3.05, 43.605) -> (-3.05, 36.3879) projected
  arc A212 (-3.05, 36.3879) -> (-3.05, 31.3679) centre (0, 33.8779) ccw projected
  line L163 (-3.05, 31.3679) -> (-3.05, 24.1507) projected
  arc A213 (-3.05, 24.1507) -> (3.05, 24.1507) centre (0, 33.8779) ccw projected
  circle A214 centre (0, 33.8779) radius 13.8038 projected
  line L164 (0, -16.8507) -> (108.7886, -16.8507)
  line L165 (108.7886, 50.7286) -> (0, 50.7286)
  line L166 (-16.8507, 0) -> (-16.8507, 33.8779)
  line L167 (125.6393, 0) -> (125.6393, 33.8779)
  constraints: 16 end point, 16 point on circle, 13 centre point, 4 vertical, 3 tangent, 2 coincident, 1 parallel, 10 other
extrude "Выдавливание2" add sketch "Эскиз2" against normal blind 5 contours A1 | A44 | A47 | A46 | A45 | A1 L165 A49 L167 A48 L164 A43 L166 | A43 | A49 | A48
